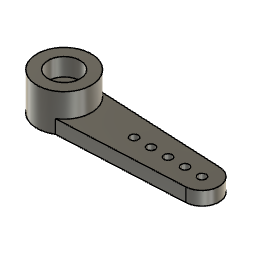
サーボホーン2 v2 (Autodesk Fusion 360 design; units mm, degrees)
Autodesk Fusion 360 part; units mm, degrees
sketch "スケッチ1" plane through (0, 0, 0) normal (0, 0, 1) x (1, 0, 0)
  line L0 (2.1071, 3.4) -> (-2.1071, 3.4) construction
  line L1 (-2.1071, -3.4) -> (2.1071, -3.4) construction
  line L2 (22.8, 3.4) -> (-22.8, 3.4) construction
  line L3 (-22.8, 3.4) -> (-22.8, -3.4) construction
  line L4 (-22.8, -3.4) -> (22.8, -3.4) construction
  line L5 (22.8, -3.4) -> (22.8, 3.4) construction
  line L6 (22.8, 3.4) -> (-22.8, -3.4) construction
  line L7 (-22.8, 3.4) -> (22.8, -3.4) construction
  line L8 (-2.1071, 3.4) -> (-20.4231, 2.497)
  line L9 (-2.1071, -3.4) -> (-20.4231, -2.497)
  line L10 (2.1071, 3.4) -> (20.4231, 2.497)
  line L11 (2.1071, -3.4) -> (20.4231, -2.497)
  arc A0 (-20.4231, 2.497) -> (-20.4231, -2.497) centre (-20.3, 0) ccw
  arc A1 (20.4231, -2.497) -> (20.4231, 2.497) centre (20.3, 0) ccw
  arc A2 (2.1071, 3.4) -> (-2.1071, 3.4) centre (0, 0) ccw
  arc A3 (-2.1071, 3.4) -> (-2.1071, -3.4) centre (0, 0) ccw
  arc A4 (2.1071, -3.4) -> (2.1071, 3.4) centre (0, 0) ccw
  arc A5 (-2.1071, -3.4) -> (2.1071, -3.4) centre (0, 0) ccw
  line L12 (-2.1071, 3.4) -> (2.1071, 3.4)
  line L13 (-2.1071, -3.4) -> (2.1071, -3.4)
  circle A6 centre (-20.3, 0) radius 0.6
  circle A7 centre (-17.8, 0) radius 0.6
  circle A8 centre (-15.3, 0) radius 0.6
  circle A9 centre (-12.8, 0) radius 0.6
  circle A10 centre (-10.3, 0) radius 0.6
  line L14 (0, 1.75) -> (0, 22.5) construction
  circle A11 centre (10.3, 0) radius 0.6
  circle A12 centre (12.8, 0) radius 0.6
  circle A13 centre (15.3, 0) radius 0.6
  circle A14 centre (17.8, 0) radius 0.6
  circle A15 centre (20.3, 0) radius 0.6
  dimension "d1" = 8
  dimension "d5" = 6.8
  dimension "d6" = 45.6
  dimension "d7" = 6.8
  dimension "d8" = 2.5
  dimension "d9" = 2.5
  dimension "d10" = 1.2
  dimension "d11" = 2.5
  dimension "d14" = 2.5
  dimension "d15" = 0
  dimension "d16" = 10
  constraint coincident A2.centre A3.centre
  constraint horizontal L0
  constraint parallel L0 L1
  constraint coincident L1.end A3
  constraint horizontal L2
  constraint perpendicular L2 L3
  constraint parallel L2 L4
  constraint parallel L3 L5
  constraint coincident L6 A2.centre
  constraint coincident L7 A2.centre
  constraint tangent L9 A0
  constraint tangent L10 A1
  constraint tangent L5 A1
  constraint tangent L11 A1
  constraint tangent L3 A0
  constraint tangent L8 A0
  constraint midpoint L3 A0
  constraint midpoint L5 A1
  constraint concentric A2 A3
  constraint concentric A3 A4
  constraint concentric A3 A5
  constraint concentric A0 A6
  constraint symmetric A6 L14 A15
  constraint symmetric A7 L14 A14
  constraint symmetric A8 L14 A13
  constraint symmetric A9 L14 A12
  constraint symmetric A10 L14 A11
  measures "d1" diameter of A3
  measures "d5" distance of L0 L1
  measures "d6" distance of L3.end L4.end
  measures "d7" distance of L2.end L3.end
  measures "d8" radius of A0
  measures "d9" radius of A1
  measures "d10" diameter of A6
  measures "d11" distance of L3 A0.centre
  measures "d16" distance of A0.centre A10.centre
extrude "押し出し1" add sketch "スケッチ1" along normal blind 5.5 contours A3 A4 L12 L13 | A2 L12 | A5 L13 makes body 1
extrude "押し出し2" add sketch "スケッチ1" along normal blind 2 contours L8 L9 A0 A3 | L10 L11 A1 A4 bodies 1
sketch "スケッチ2" plane through (0, 0, 5.5) normal (0, 0, 1) x (-1, 0, 0)
  circle A0 centre (0, 0) radius 4
  circle A1 centre (0, 0) radius 1
  circle A2 centre (0, 0) radius 2.35
  dimension "d23" = 2
  dimension "d24" = 4.7
  constraint coincident A0.centre A1.centre
  measures "d23" diameter of A1
  measures "d24" diameter of A2
extrude "押し出し3" cut sketch "スケッチ2" against normal through all contours A1 bodies 1
extrude "押し出し4" cut sketch "スケッチ2" against normal blind 2.6 contours A2 bodies 1
sketch "スケッチ3" plane through (0, 0, 0) normal (0, 0, 1) x (1, 0, 0)
  circle A0 centre (0, 0) radius 3.1
  dimension "d28" = 6.2
  constraint coincident A0.centre origin
  measures "d28" diameter of A0
extrude "押し出し5" cut sketch "スケッチ3" along normal blind 2.1 bodies 1
copy_body "ボディ -> コンポーネント1" bodies 1 removing the originals makes body 2 in component "Component'"
split "分割1" by face at (1.6962, 3.6226, 2.5) of body 2 bodies 2 makes body 3 at (11.7618, -2.1651, 2) makes body 4 at (-11.7618, -2.1651, 0) in component "Component'"
delete_body "RemoveBody1" bodies 4 in component "Component'"
combine "結合1" operation add target body 2 tool bodies 3 in component "Component'"
component "Component'" placed x (1, 0, 0) y (0, 1, 0) z (0, 0, 1) at (0, 0, 0)
